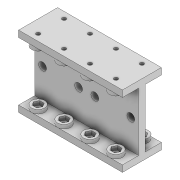
# Autodesk Inventor part: ExtConnector
Saved by Autodesk Inventor 2022 (Build 260153000, 153)
## iProperties
Created: 2022-10-27
Part Number: ExtConnector
Material: Generic
Document SubType Name: Modeling
Designer: MVeszpremi
Density: 1 g/cm^3
Appearance: Default
Author: MVeszpremi
Autodesk Inventor part; units mm, degrees
ref_plane "YZ Plane" through (0, 0, 0) normal (1, 0, 0) x (0, 1, 0)
sketch "Sketch1" plane through (0, 0, 0) normal (0, 0, 1) x (1, 0, 0)
  line L0 (0, 0) -> (100, 0)
  line L1 (100, 0) -> (100, 55)
  line L2 (100, 55) -> (0, 55)
  line L3 (0, 55) -> (0, 0)
  dimension "d0" = 55
  dimension "d1" = 100
  constraints: 8 end point, 2 parallel, 1 horizontal, 1 perpendicular
  measures "d0" distance of L2.end L0.start
  measures "d1" distance of L1.end L2.end
extrude "Extrusion1" add sketch "Sketch1" along normal blind 5
sketch "Sketch2" plane through (0, 0, 5) normal (0, 0, 1) x (1, 0, 0)
  line L0 (0, 55) -> (0, 0) projected
  line L1 (100, 0) -> (100, 55) projected
  line L2 (0, 0) -> (100, 0)
  line L3 (100, 0) -> (100, 5)
  line L4 (100, 5) -> (0, 5)
  line L5 (0, 5) -> (0, 0)
  point P0 (0, 5)
  dimension "d4" = 5
  constraints: 8 end point, 2 parallel, 1 horizontal, 1 perpendicular, 1 point on line
  measures "d4" distance between parallel lines of L2 L4
extrude "Extrusion2" add sketch "Sketch2" along normal blind 12.5
sketch "Sketch3" plane through (0, 5, 5) normal (0, 1, 0) x (1, 0, 0)
  line L0 (100, 0) -> (0, 0) projected
  line L1 (50, 0) -> (50, -12.5)
  line L2 (0, -12.5) -> (100, -12.5) projected
  circle A0 centre (30, -7.5) radius 1.5
  line L3 (0, 0) -> (0, -12.5) projected
  point P0 (0, 5)
  dimension "d8" = 3
  dimension "d33" = 30
  dimension "d34" = 7.5
  constraints: 2 end point, 2 midpoint, 1 centre point
  measures "d8" diameter of A0
  measures "d33" horizontal distance of L2.start A0.centre
  measures "d34" distance from line of L0 A0.centre
extrude "Extrusion3" cut sketch "Sketch3" against normal blind 12.5 contours A0
pattern_linear "Rectangular Pattern1" count 4 spacing 20 along (1, 0, 0) of "Extrusion3"
sketch "Sketch4" plane through (0, 5, 5) normal (0, 1, 0) x (1, 0, 0)
  circle A0 centre (30, -7.5) radius 1.5 projected
  line L0 (26.5359, -7.5) -> (28.2679, -4.5)
  line L1 (28.2679, -4.5) -> (31.7321, -4.5)
  line L2 (31.7321, -4.5) -> (33.4641, -7.5)
  line L3 (33.4641, -7.5) -> (31.7321, -10.5)
  line L4 (31.7321, -10.5) -> (28.2679, -10.5)
  line L5 (28.2679, -10.5) -> (26.5359, -7.5)
  circle A1 centre (30, -7.5) radius 5
  point P0 (0, 5)
  dimension "d14" = 6
  constraints: 12 end point, 2 coincident, 1 centre point, 13 other
  measures "d14" distance between parallel lines of L1 L4
extrude "Extrusion4" add sketch "Sketch4" along normal blind 3 contours A1
pattern_linear "Rectangular Pattern2" count 4 spacing 20 along (1, 0, 0) of "Extrusion4"
ref_plane "Work Plane1" through (0, 0, 2.5) normal (0, 0, 1) x (1, 0, 0)
mirror "Mirror1" about plane through (0, 0, 2.5) normal (0, 0, 1) of "Extrusion4", "Rectangular Pattern2", "Extrusion3", "Rectangular Pattern1", "Extrusion2"
ref_plane "Work Plane3" through (0, 27.5, 0) normal (0, 1, 0) x (1, 0, 0)
mirror "Mirror3" about plane through (0, 27.5, 0) normal (0, 1, 0) of "Extrusion4", "Rectangular Pattern2", "Extrusion3", "Rectangular Pattern1", "Extrusion2", "Mirror1"
sketch "Sketch6" plane through (0, 5, 5) normal (0, 1, 0) x (1, 0, 0)
  line L0 (0, 5) -> (0, 17.5) projected
  line L1 (0, -12.5) -> (100, -12.5) projected
  line L2 (0, 17.5) -> (20, 17.5)
  line L3 (20, 17.5) -> (20, -12.5)
  line L4 (20, -12.5) -> (0, -12.5)
  line L5 (0, -12.5) -> (0, 17.5)
  line L6 (0, 5) -> (20, 5)
  line L7 (20, 5) -> (20, 0)
  line L8 (20, 0) -> (0, 0)
  line L9 (0, 0) -> (0, 5)
  point P0 (0, -12.5)
  dimension "d21" = 20
  constraints: 16 end point, 4 parallel, 2 horizontal, 2 perpendicular, 2 point on line
  measures "d21" distance between parallel lines of L0 L3
extrude "Extrusion5" cut sketch "Sketch6" along normal blind 53.5 and the other way blind 13.5
sketch "Sketch8" plane through (0, 0, 5) normal (0, 0, 1) x (1, 0, 0)
  circle A0 centre (26, 27.5) radius 3
  circle A1 centre (53.75, 27.5) radius 3
  circle A2 centre (66.25, 27.5) radius 3
  circle A3 centre (94, 27.5) radius 3
  line L0 (20, 5) -> (20, 50) projected
  line L1 (20, 27.5) -> (100, 27.5)
  line L2 (100, 5) -> (100, 50) projected
  point P0 (0, 0)
  dimension "d35" = 6
  dimension "d36" = 6
  dimension "d37" = 6
  dimension "d38" = 6
  dimension "d39" = 6
  dimension "d40" = 12.5
  dimension "d41" = 33.75
  dimension "d42" = 6
  constraints: 4 centre point, 4 point on line, 2 end point, 2 midpoint
  measures "d35" diameter of A0
  measures "d36" diameter of A1
  measures "d37" diameter of A2
  measures "d38" diameter of A3
  measures "d39" distance of L1.start A0.centre
  measures "d40" distance of A2.centre A1.centre
  measures "d41" distance from line of L0 A1.centre
  measures "d42" distance from line of L2 A3.centre
extrude "Extrusion7" cut sketch "Sketch8" against normal blind 10
body "Solid1"
